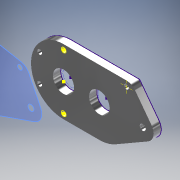
# Autodesk Inventor part: Inner Plate
Saved by Autodesk Inventor 2019.4 (Build 234330000, 330)
## iProperties
Created: 2019-12-31
Part Number: Inner Plate
Material: Aluminum 6061
Document SubType Name: Modeling
Designer: Mark
Mass: 80.5102 g
Surface Area: 120.39 cm^2
Volume: 29.8186 cm^3
Density: 2.7 g/cm^3
Appearance: Aluminum - Flat
Author: Mark
Autodesk Inventor part; units mm, degrees
ref_plane "YZ Plane" through (0, 0, 0) normal (1, 0, 0) x (0, 1, 0)
ref_plane "XZ Plane" through (0, 0, 0) normal (0, 1, 0) x (-1, 0, 0)
ref_plane "XY Plane" through (0, 0, 0) normal (0, 0, 1) x (1, 0, 0)
sketch "Sketch1" plane through (0, 0, 0) normal (0, 0, 1) x (1, 0, 0)
  circle A0 centre (0, 0) radius 7.62 construction
  circle A1 centre (0, 0) radius 9.75
  circle A2 centre (33.02, 0) radius 25.4 construction
  line L0 (0, 0) -> (7.62, 0)
  line L1 (0, 0) -> (7.62, 0) construction
  circle A3 centre (33.02, 0) radius 9.5
  line L2 (0, -30) -> (33.02, -30)
  line L3 (33.02, 30) -> (0, 30)
  arc A4 (33.02, -30) -> (63.02, 0) centre (33.02, 0) ccw
  arc A5 (0, 30) -> (0, -30) centre (0, 0) ccw
  circle A6 centre (0, 0) radius 25.4 construction
  line L4 (0, 25.4) -> (0, 0) construction
  line L5 (0, 25.4) -> (25.4, 25.4) construction
  circle A7 centre (0, 25.4) radius 2.2
  circle A8 centre (-21.997, 12.7) radius 2.2
  circle A9 centre (-21.997, -12.7) radius 2.2
  circle A10 centre (0, -25.4) radius 2.2
  circle A11 centre (21.997, -12.7) radius 2.2
  circle A12 centre (21.997, 12.7) radius 2.2
  line L6 (63.02, 0) -> (63.02, 30)
  line L7 (63.02, 30) -> (33.02, 30)
  circle A13 centre (58.02, 25) radius 2.2
  circle A14 centre (73.02, 0) radius 2.75
  circle A15 centre (73.02, 0) radius 10
  line L8 (81.02, 6) -> (63.02, 30)
  line L9 (78.02, -8.6603) -> (48.02, -25.9808)
  dimension "d13" = 50.8
  dimension "d0" = 15.24
  dimension "d1" = 19.5
  dimension "d2" = 50.8
  dimension "d3" = 7.62
  dimension "d4" = 0
  dimension "d5" = 33.02
  dimension "d6" = 19
  dimension "d9" = 30
  dimension "d10" = 60
  dimension "d14" = 25.4
  dimension "d15" = 90
  dimension "d16" = 4.4
  dimension "d19" = 360
  dimension "d21" = 30
  dimension "d22" = 30
  dimension "d26" = 90
  dimension "d28" = 4.4
  dimension "d29" = 5
  dimension "d30" = 5
  dimension "d38" = 5.5
  dimension "d39" = 10
  dimension "d40" = 20
  constraints: 20 end point, 15 centre point, 11 coincident, 7 point on circle, 4 horizontal, 4 tangent, 2 equal length, 2 parallel, 2 point on line, 1 equal radius, 1 perpendicular, 1 vertical alignment, 15 other
  measures "d0" diameter of A0
  measures "d1" diameter of A1
  measures "d2" diameter of A2
  measures "d3" distance of L0.start L0.end
  measures "d4" distance between parallel lines of L0 L1
  measures "d5" distance of A2.centre L0.start
  measures "d6" diameter of A3
  measures "d9" radius of A4
  measures "d10" distance between parallel lines of L3 L2
  measures "d14" distance of L4.start L4.end
  measures "d15" angle of L4 L5
  measures "d16" diameter of A7
  measures "d21" distance of L3.start L6.end
  measures "d22" distance of L6.start L6.end
  measures "d26" angle of L0 L6
  measures "d28" diameter of A13
  measures "d29" distance from line of L7 A13.centre
  measures "d30" distance from line of L6 A13.centre
  measures "d38" diameter of A14
  measures "d39" distance from line of L6 A14.centre
  measures "d40" diameter of A15
extrude "Extrusion1" add sketch "Sketch1" along normal blind 7 contours A5 L3 L7 L6 A4 L2 | A4 A15 L9 | L6 L8 A15 | A15 | A11 | A12
fillet "Fillet2" radius 10 1 edges at (63.02, 30, 3.5)
body "Solid1"
